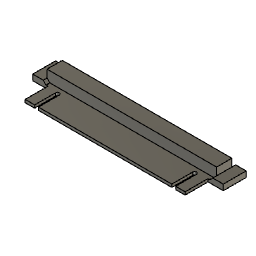
Comb v2 (Autodesk Fusion 360 design; units mm, degrees)
Autodesk Fusion 360 part; units mm, degrees
sketch "Sketch1" plane through (0, 0, 0) normal (0, 0, 1) x (1, 0, 0) in component "Comb"
  line L0 (0, 0) -> (-50, 0)
  line L1 (0, 0) -> (50, 0)
  line L2 (50, 0) -> (50, 20)
  line L3 (50, 20) -> (-50, 20)
  line L4 (-50, 20) -> (-50, 0)
  line L5 (0, -20) -> (30, -20)
  line L6 (35, -20) -> (45, -20)
  line L7 (45, -20) -> (45, 0)
  line L8 (35, -20) -> (35, 0)
  line L9 (30, -20) -> (30, 0)
  line L10 (-45, -20) -> (-45, 0)
  line L11 (-30, -20) -> (-30, 0)
  line L12 (-35, -20) -> (-35, 0)
  line L13 (0, -20) -> (-30, -20)
  line L14 (-35, -20) -> (-45, -20)
  dimension "d3" = 20
  dimension "d4" = 100
  constraint coincident L0.start L1.start
  constraint coincident L1 L7.end
  constraint coincident L1 L8.end
  constraint coincident L1 L9.end
  measures "d3" distance of L1.end L2.end
  measures "d4" distance of L2.end L3.end
extrude "Extrude1" add sketch "Sketch1" along normal blind 20 contours L0 L1 L2 L3 L4 makes body 1 in component "Comb"
extrude "Extrude2" add sketch "Sketch1" along normal blind 1 contours L0 L1 L5 L9 L11 L13 | L0 L10 L12 L14 | L1 L6 L7 L8 bodies 1 in component "Comb"
sketch "Sketch2" plane through (0, 0, 0) normal (0, 0, 1) x (1, 0, 0) in component "Comb"
  line L0 (0, 0) -> (42, 0)
  line L1 (42, 0) -> (42, -12)
  line L2 (42, -12) -> (37, -12)
  line L3 (37, -12) -> (37, 0)
  line L4 (0, -12) -> (35, -12)
  line L5 (35, -12) -> (35, 0)
  line L6 (42, 0) -> (50, 0)
  line L7 (50, 0) -> (50, 12)
  line L8 (50, 12) -> (0, 12)
  line L9 (-42, 0) -> (-42, -12)
  line L10 (-35, -12) -> (-35, 0)
  line L11 (-50, 0) -> (-50, 12)
  line L12 (-50, 12) -> (0, 12)
  line L13 (0, -12) -> (-35, -12)
  line L14 (-42, -12) -> (-37, -12)
  line L15 (0, 0) -> (-42, 0)
  line L16 (-42, 0) -> (-50, 0)
  line L17 (-37, -12) -> (-37, 0)
  line L18 (0, 0) -> (0, 2)
  line L19 (0, 10) -> (44.5, 10)
  line L20 (0, 2) -> (44.5, 2)
  line L21 (44.5, 2) -> (44.5, 10)
  line L22 (44.5, 2) -> (44.5, 0)
  line L23 (44.5, 10) -> (44.5, 12)
  line L24 (-44.5, 10) -> (-44.5, 12)
  line L25 (-44.5, 2) -> (-44.5, 10)
  line L26 (-44.5, 2) -> (-44.5, 0)
  line L27 (0, 2) -> (-44.5, 2)
  line L28 (0, 10) -> (-44.5, 10)
  dimension "d13" = 12
  dimension "d14" = 42
  dimension "d16" = 5
  dimension "d17" = 35
  dimension "d19" = 12
  dimension "d20" = 50
  dimension "d25" = 2
  dimension "d26" = 2
  dimension "d27" = 44.5
  dimension "d28" = 44.5
  constraint coincident L0.start L15.start
  constraint coincident L0 L3.end
  constraint coincident L0 L5.end
  constraint coincident L6 L22.end
  constraint coincident L8 L23.end
  measures "d13" distance of L0.start L4.start
  measures "d14" distance of L0.start L0.end
  measures "d16" distance of L1.end L2.end
  measures "d17" distance of L4.start L4.end
  measures "d19" distance of L6.end L7.end
  measures "d20" distance of L7.end L8.end
  measures "d25" distance of L0.start L18.end
  measures "d26" distance of L8.end L19.start
  measures "d27" distance of L19.start L19.end
  measures "d28" distance of L18.end L20.end
extrude "Extrude3" add sketch "Sketch2" along normal blind 1 separate body contours L0 L4 L5 L10 L13 L15 | L0 L1 L2 L3 | L9 L14 L15 L17 makes body 2 at (-11.6667, -4, 0) makes body 3 at (38.6667, -4, 0) makes body 4 at (-40.3333, -4, 0) in component "Comb"
extrude "Extrude4" add sketch "Sketch2" along normal blind 1 contours L0 L6 L18 L20 L22 | L15 L16 L18 L26 L27 | L19 L20 L21 L25 L27 L28 | L6 L7 L8 L21 L22 L23 | L11 L12 L16 L24 L25 L26 | L8 L12 L19 L23 L24 L28 bodies 2 3 4 in component "Comb"
extrude "Extrude5" add sketch "Sketch2" along normal blind 3 contours L6 L7 L8 L21 L22 L23 | L11 L12 L16 L24 L25 L26 bodies 2 in component "Comb"
extrude "Extrude6" add sketch "Sketch2" along normal blind 7 contours L19 L20 L21 L25 L27 L28 bodies 2 in component "Comb"
chamfer "Chamfer1" distance 2 angle 45 4 edges at (-44.5, 1, 1) (44.5, 1, 1) (44.5, 11, 1) (-44.5, 11, 1) on bodies 2 in component "Comb"
fillet "Fillet1" radius 1 4 edges at (-37, 0, 0.5) (-35, 0, 0.5) (37, 0, 0.5) (35, 0, 0.5) on bodies 2 in component "Comb"
delete_body "RemoveBody1" bodies 1 in component "Comb"
copy_body "CopyPasteBodies1" bodies 2 makes body 5 in component "Comb"
extrude "Extrude7" cut 1 faces at (-11.6667, -4.6665, 1) along direction (0, 0, -1) blind 0.5 on bodies 5 bodies 5 in component "Comb"
extrude "Extrude8" add sketch "Sketch2" along normal blind 1 separate body makes body 6 in component "Comb"
copy_body "CopyPasteBodies2" bodies 2 makes body 7 in component "Comb"
move_face "OffsetFaces1" offset 0.5 1 faces at (-11.6667, -4.6665, 1) on bodies 7 in component "Comb"
component "Comb" placed x (1, 0, 0) y (0, 1, 0) z (0, 0, 1) at (0, 0, 0)
hidden bodies 2 5 6
equation "d27 = ( 89 / 2 ) * 1 mm"
equation "d28 = ( 89 / 2 ) * 1 mm"
named bodies: "Comb", "Comb Thin", "Comb Flat", "Comb (1)", "Comb 1.5mm"
